duplicate (Autodesk Fusion 360 design; units mm, degrees)
Autodesk Fusion 360 part; units mm, degrees
sketch "Sketch2" plane through (0, 0, 0) normal (0, 1, 0) x (1, 0, 0) in component "oldroom"
  line L0 (0, 0) -> (2909, 0)
  line L1 (2909, 0) -> (2909, -3651)
  line L2 (2909, -3651) -> (0, -3651)
  line L3 (0, -3651) -> (0, 0)
  line L4 (2909, 0) -> (1648, 0)
  line L5 (1648, 0) -> (1648, -944)
  line L6 (1648, -944) -> (2909, -944)
  line L7 (2909, -944) -> (2909, 0)
  constraint horizontal L0
  constraint vertical L1
  constraint horizontal L2
  constraint vertical L3
  constraint coincident L0.start L3.end
  constraint horizontal L4
  constraint vertical L5
  constraint horizontal L6
  constraint vertical L7
extrude "Extrude1" add sketch "Sketch2" against normal blind 100 makes body 1 in component "walls"
extrude "Extrude2" add sketch "Sketch2" along normal blind 2405 contours L0 L1 L4 L5 L6 L7 bodies 1 in component "walls"
sketch "Sketch1" plane through (0, 0, 0) normal (0, 0, 1) x (1, 0, 0) in component "walls"
  line L0 (0, 0) -> (2909, 0)
  line L1 (2909, 0) -> (2909, 2405)
  line L2 (2909, 2405) -> (0, 2405)
  line L3 (0, 2405) -> (0, 0)
  line L4 (2909, -100) -> (2909, 2405)
  line L5 (2909, 0) -> (2909, 2405)
  constraint horizontal L0
  constraint vertical L1
  constraint horizontal L2
  constraint vertical L3
  constraint coincident L1.end L4
  constraint coincident L0.start L3.end
sketch "Sketch2 (2)" plane through (0, 0, 0) normal (1, 0, 0) x (0, 0, -1) in component "walls"
  line L0 (0, 0) -> (-3651, 0)
  line L1 (-3651, 0) -> (-3651, 2405)
  line L2 (-3651, 2405) -> (0, 2405)
  line L3 (0, 2405) -> (0, 0)
  constraint horizontal L0
  constraint vertical L1
  constraint horizontal L2
  constraint vertical L3
  constraint coincident L0.start L3.end
sketch "Sketch3" plane through (1648, 0, 0) normal (-1, 0, 0) x (0, 0, 1) in component "walls"
  line L0 (0, 0) -> (944, 0)
  line L1 (944, 0) -> (944, 2405)
  line L2 (944, 2405) -> (0, 2405)
  line L3 (0, 2405) -> (0, 0)
  line L4 (100, 0) -> (862, 0)
  line L5 (862, 0) -> (862, 1879.6)
  line L6 (862, 1879.6) -> (100, 1879.6)
  line L7 (100, 1879.6) -> (100, 0)
  constraint horizontal L4
  constraint vertical L5
  constraint horizontal L6
  constraint vertical L7
sketch "Sketch1 (2)" plane through (1648, 939.8, 481) normal (-1, 0, 0) x (0, 0, 1) in component "door"
extrude "Extrude1'" add sketch "Sketch3" against normal blind 35 separate body contours L0 L4 L5 L6 L7 makes body 2 in component "door"
sketch "Sketch1 (3)" plane through (0, 0, 0) normal (0, 1, 0) x (1, 0, 0) in component "shelving"
  line L0 (0, 0) -> (410, 0)
  line L1 (410, 0) -> (410, -910)
  line L2 (410, -910) -> (0, -910)
  line L3 (0, -910) -> (0, 0)
  constraint horizontal L0
  constraint vertical L1
  constraint horizontal L2
  constraint vertical L3
  constraint coincident L0.start L3.end
extrude "Extrude1''" add sketch "Sketch1 (3)" along normal blind 1830 separate body makes body 3 in component "shelving"
sketch "Sketch1 (4)" plane through (0, 0, 0) normal (0, 1, 0) x (1, 0, 0) in component "bed"
  line L0 (0, 0) -> (910, 0)
  line L1 (910, 0) -> (910, -1900)
  line L2 (910, -1900) -> (0, -1900)
  line L3 (0, -1900) -> (0, 0)
  constraint horizontal L0
  constraint vertical L1
  constraint horizontal L2
  constraint vertical L3
  constraint coincident L0.start L3.end
extrude "Extrude1'''" add sketch "Sketch1 (4)" along normal blind 800 separate body makes body 4 in component "bed"
move_body "Align1" bodies 4 to x (1, 0, 0) y (0, 1, 0) z (0, 0, 1) at (-146, 0, 0) in component "bed"
move_body "Align2" bodies 4 to x (1, 0, 0) y (0, 1, 0) z (0, 0, 1) at (0, 0, 4) in component "bed"
sketch "Sketch1 (5)" plane through (0, 0, 0) normal (0, 1, 0) x (1, 0, 0) in component "junk boxes"
  line L0 (2909, -3651) -> (1009, -3651)
  line L1 (1009, -3651) -> (1009, -2251)
  line L2 (1009, -2251) -> (2909, -2251)
  line L3 (2909, -2251) -> (2909, -3651)
  point P0 (2909, -3651)
  constraint horizontal L0
  constraint vertical L1
  constraint horizontal L2
  constraint vertical L3
  constraint coincident P0 L0.start
extrude "Extrude1''''" add sketch "Sketch1 (5)" along normal blind 200 separate body makes body 5 in component "junk boxes"
move_body "Align1'" bodies 3 to x (1, 0, 0) y (0, 1, 0) z (0, 0, 1) at (-31, 0, 0) in component "shelving"
move_face "MoveFace1" by (0, 0, -950) 1 faces at (2275.6667, 66.6667, 3651) on bodies 5 in component "junk boxes"
move_face "MoveFace2" by (0, 800, 0) 1 faces at (2275.6667, 200, 2551) on bodies 5 in component "junk boxes"
move_face "MoveFace3" by (1000, 0, 0) 1 faces at (1009, 333.3333, 2551) on bodies 5 in component "junk boxes"
sketch "Sketch1 (6)" plane through (0, 0, 0) normal (0, 1, 0) x (1, 0, 0) in component "computer table"
  line L0 (2909, -944) -> (2179, -944)
  line L1 (2179, -944) -> (2179, -1800)
  line L2 (2179, -1800) -> (2909, -1800)
  line L3 (2909, -1800) -> (2909, -944)
  point P0 (2909, -944)
  constraint horizontal L0
  constraint vertical L1
  constraint horizontal L2
  constraint vertical L3
  constraint coincident P0 L0.start
extrude "Extrude1'''''" add sketch "Sketch1 (6)" along normal blind 730 separate body makes body 6 in component "computer table"
sketch "Sketch1 (7)" plane through (0, 0, 0) normal (0, 1, 0) x (1, 0, 0) in component "chair"
  line L0 (1000, -1100) -> (1510, -1100)
  line L1 (1510, -1100) -> (1510, -1670)
  line L2 (1510, -1670) -> (1000, -1670)
  line L3 (1000, -1670) -> (1000, -1100)
  constraint horizontal L0
  constraint vertical L1
  constraint horizontal L2
  constraint vertical L3
extrude "Extrude1''''''" add sketch "Sketch1 (7)" along normal blind 560 separate body makes body 7 in component "chair"
sketch "Sketch2 (3)" plane through (0, 560, 0) normal (0, 1, 0) x (-1, 0, 0) in component "chair"
  line L0 (-1000, 1670) -> (-1510, 1670)
  line L1 (-1510, 1670) -> (-1510, 1100)
  line L2 (-1510, 1100) -> (-1000, 1100)
  line L3 (-1000, 1100) -> (-1000, 1670)
  line L4 (-1000, 1100) -> (-900, 1100)
  line L5 (-900, 1100) -> (-900, 1670)
  line L6 (-900, 1670) -> (-1000, 1670)
  line L7 (-1000, 1670) -> (-1000, 1100)
  constraint horizontal L4
  constraint vertical L5
  constraint horizontal L6
  constraint vertical L7
  constraint coincident L2.end L3.start
extrude "Extrude2'" add sketch "Sketch2 (3)" along normal blind 590 separate body contours L3 L4 L5 L6 L7 makes body 8 in component "chair"
sketch "Sketch1 (8)" plane through (0, 0, 0) normal (0, 1, 0) x (1, 0, 0) in component "small chest of draws"
  line L0 (0, -3651) -> (634.8984, -3651)
  line L1 (634.8984, -3651) -> (634.8984, -3214.5264)
  line L2 (634.8984, -3214.5264) -> (0, -3214.5264)
  line L3 (0, -3214.5264) -> (0, -3651)
  point P0 (0, -3651)
  constraint horizontal L0
  constraint vertical L1
  constraint horizontal L2
  constraint vertical L3
  constraint coincident P0 L0.start
extrude "Extrude1'''''''" add sketch "Sketch1 (8)" along normal blind 666.9024 separate body makes body 9 in component "small chest of draws"
sketch "Sketch1 (9)" plane through (0, 0, 0) normal (0, 1, 0) x (1, 0, 0) in component "wooden shelving"
  line L0 (0, 0) -> (500, 0)
  line L1 (500, 0) -> (500, -812)
  line L2 (500, -812) -> (0, -812)
  line L3 (0, -812) -> (0, 0)
  constraint horizontal L0
  constraint vertical L1
  constraint horizontal L2
  constraint vertical L3
  constraint coincident L0.start L3.end
extrude "Extrude1''''''''" add sketch "Sketch1 (9)" along normal blind 1800 separate body makes body 10 in component "wooden shelving"
sketch "Sketch1 (10)" plane through (0, 0, 0) normal (0, 1, 0) x (1, 0, 0) in component "chest of draws"
  line L0 (0, -800) -> (500, -800)
  line L1 (500, -800) -> (500, -1416)
  line L2 (500, -1416) -> (0, -1416)
  line L3 (0, -1416) -> (0, -800)
  constraint horizontal L0
  constraint vertical L1
  constraint horizontal L2
  constraint vertical L3
extrude "Extrude1'''''''''" add sketch "Sketch1 (10)" along normal blind 1300 separate body makes body 11 in component "chest of draws"
sketch "Sketch1 (11)" plane through (0, 0, 0) normal (0, 1, 0) x (1, 0, 0) in component "hollow stand"
  line L0 (0, -1416) -> (500, -1416)
  line L1 (500, -1416) -> (500, -2516)
  line L2 (500, -2516) -> (0, -2516)
  line L3 (0, -2516) -> (0, -1416)
  point P0 (0, -1416)
  constraint horizontal L0
  constraint vertical L1
  constraint horizontal L2
  constraint vertical L3
  constraint coincident P0 L0.start
extrude "Extrude1''''''''''" add sketch "Sketch1 (11)" along normal blind 910 separate body makes body 12 in component "hollow stand"
move_body "Align1''" bodies 11 to x (1, 0, 0) y (0, 1, 0) z (0, 0, 1) at (0, 0, 12) in component "chest of draws"
move_body "Align2'" bodies 11 to x (1, 0, 0) y (0, 1, 0) z (0, 0, 1) at (0, 0, -190) in component "chest of draws"
move_body "Align1'''" bodies 12 to x (1, 0, 0) y (0, 1, 0) z (0, 0, 1) at (0, 0, 12) in component "hollow stand"
move_body "Align2''" bodies 12 to x (1, 0, 0) y (0, 1, 0) z (0, 0, 1) at (0, 0, 0) in component "hollow stand"
move_body "Align3" bodies 12 to x (1, 0, 0) y (0, 1, 0) z (0, 0, 1) at (0, 0, -70) in component "hollow stand"
sketch "Sketch1 (12)" plane through (0, 0, 0) normal (0, 1, 0) x (1, 0, 0) in component "bed (1)"
  line L0 (0, 0) -> (910, 0)
  line L1 (910, 0) -> (910, -1900)
  line L2 (910, -1900) -> (0, -1900)
  line L3 (0, -1900) -> (0, 0)
  constraint horizontal L0
  constraint vertical L1
  constraint horizontal L2
  constraint vertical L3
  constraint coincident L0.start L3.end
extrude "Extrude1'''''''''''" add sketch "Sketch1 (12)" along normal blind 800 separate body makes body 13 in component "bed (1)"
move_body "Align1''''" bodies 13 to x (1, 0, 0) y (0, 1, 0) z (0, 0, 1) at (-146, 0, 0) in component "bed (1)"
move_body "Align2'''" bodies 13 to x (1, 0, 0) y (0, 1, 0) z (0, 0, 1) at (0, 0, 4) in component "bed (1)"
extrude "Extrude1''''''''''''" add 1 faces at (157.3333, 800, 1270.6667) faces seen with x (0, 0, -1) y (0, 1, 0) z (1, 0, 0) at (1005, 0, 3505) along direction (0, -1, 0) blind 800 separate body on bodies 13 makes body 14 in component "newroom"
extrude "Extrude2''" cut 1 faces at (2275.6667, 800, 3347.6667) along direction (0, -1, 0) blind 550 on bodies 14 bodies 14 in component "newroom"
sketch "Sketch1 (13)" plane through (0, -300, 0) normal (0, 1, 0) x (-1, 0, 0) in component "desk 1"
  line L0 (-1009, 4002.0003) -> (-65, 4002.0003)
  line L1 (-65, 4002.0003) -> (-65, 5650.0003)
  line L2 (-65, 5650.0003) -> (-3716, 5650.0003)
  line L3 (-3716, 5650.0003) -> (-3716, 2741.0003)
  line L4 (-3716, 2741.0003) -> (-1009, 2741.0003)
  line L5 (-1009, 2741.0003) -> (-1009, 4002.0003)
  line L6 (-65, 5650.0003) -> (-3716, 5650.0003)
  line L7 (-3716, 5650.0003) -> (-3716, 4750.0003)
  line L8 (-3716, 4750.0003) -> (-65, 4750.0003)
  line L9 (-65, 4750.0003) -> (-65, 5650.0003)
  constraint horizontal L6
  constraint vertical L7
  constraint horizontal L8
  constraint vertical L9
  constraint coincident L3 L7.end
  constraint coincident L1.end L2.start
extrude "Extrude1'''''''''''''" add sketch "Sketch1 (13)" along normal blind 50 separate body contours L1 L2 L3 L6 L7 L8 L9 makes body 15 in component "desk 1"
copy_body "CutPasteBodies1" bodies 14 removing the originals makes body 16 in component "bed (2)"
sketch "Sketch1 (14)" plane through (65, -300, 5650.0003) normal (0, 0, -1) x (-1, 0, 0) in component "Component"
sketch "Sketch2 (4)" plane through (0, -300, 0) normal (0, 1, 0) x (-1, 0, 0) in component "Component"
  line L0 (-1009, 4002.0003) -> (-65, 4002.0003)
  line L1 (-65, 4002.0003) -> (-65, 5650.0003)
  line L2 (-65, 5650.0003) -> (-3716, 5650.0003)
  line L3 (-3716, 5650.0003) -> (-3716, 2741.0003)
  line L4 (-3716, 2741.0003) -> (-1009, 2741.0003)
  line L5 (-1009, 2741.0003) -> (-1009, 4002.0003)
sketch "Sketch1 (15)" plane through (65, -300, 5650.0003) normal (0, 0, -1) x (-1, 0, 0) in component "lcd"
  line L0 (-2955.2121, 1965.6881) -> (-2314.4721, 1965.6881)
  line L1 (-2314.4721, 1965.6881) -> (-2314.4721, 1586.0281)
  line L2 (-2314.4721, 1586.0281) -> (-2955.2121, 1586.0281)
  line L3 (-2955.2121, 1586.0281) -> (-2955.2121, 1965.6881)
  constraint horizontal L0
  constraint vertical L1
  constraint horizontal L2
  constraint vertical L3
extrude "Extrude1''''''''''''''" add sketch "Sketch1 (15)" along normal blind 51.5 separate body makes body 17 in component "lcd"
copy_body "CopyPasteBodies1" bodies 17 makes body 18 in component "lcd"
move_body "Move1" bodies 18 to x (1, 0, 0) y (0, 1, 0) z (0, 0, 1) at (-700, 0, 0) in component "lcd"
sketch "Sketch2 (5)" plane through (465, 200, 5650.0003) normal (0, 0, -1) x (-1, 0, 0) in component "lcd"
  line L0 (-1914.4721, 1465.6881) -> (-1855.2121, 1465.6881)
  line L1 (-1855.2121, 1465.6881) -> (-1855.2121, 850.1808)
  line L2 (-1855.2121, 850.1808) -> (-1914.4721, 850.1808)
  line L3 (-1914.4721, 850.1808) -> (-1914.4721, 1465.6881)
  line L4 (-1855.2121, 1359.1726) -> (-1535.2121, 1359.1726)
  line L5 (-1535.2121, 1359.1726) -> (-1535.2121, 1259.1726)
  line L6 (-1535.2121, 1259.1726) -> (-1855.2121, 1259.1726)
  line L7 (-1855.2121, 1259.1726) -> (-1855.2121, 1359.1726)
  line L8 (-1914.4721, 1359.1726) -> (-2234.4721, 1359.1726)
  line L9 (-2234.4721, 1359.1726) -> (-2234.4721, 1259.1726)
  line L10 (-2234.4721, 1259.1726) -> (-1914.4721, 1259.1726)
  line L11 (-1914.4721, 1259.1726) -> (-1914.4721, 1359.1726)
  point P0 (-1914.4721, 1465.6881)
  constraint horizontal L0
  constraint vertical L1
  constraint horizontal L2
  constraint vertical L3
  constraint coincident P0 L0.start
  constraint horizontal L4
  constraint vertical L5
  constraint horizontal L6
  constraint vertical L7
  constraint coincident L1 L4.start
  constraint horizontal L8
  constraint vertical L9
  constraint horizontal L10
  constraint vertical L11
  constraint coincident L3 L8.start
extrude "Extrude2'''" add sketch "Sketch2 (5)" along normal blind 100 separate body makes body 19 in component "lcd"
extrude "Extrude3" cut 1 faces at (2592.8054, 1492.5059, 5550.0003) along direction (0, 0, 1) blind 50 on bodies 19 bodies 17 18 19 in component "lcd"
move_body "Move2" bodies 17 18 to x (1, 0, 0) y (0, 1, 0) z (0, 0, 1) at (0, 0, -100) in component "lcd"
combine "Combine1" operation add target body 17 tool bodies 19 makes body 20 at (2592.8054, 1492.5059, 5650.0003) in component "lcd"
extrude "Extrude4" add 1 faces at (2213.5454, 1525.8393, 5500.0003) along direction (0, 0, -1) blind 1 on bodies 18 bodies 18 in component "lcd"
extrude "Extrude5" add 1 faces at (2213.5454, 1525.8393, 5499.0003) along direction (0, 0, -1) blind 0.5 on bodies 18 bodies 18 in component "lcd"
extrude "Extrude6" add 1 faces at (2592.8054, 1492.5059, 5500.0003) along direction (0, 0, -1) blind 1.5 on bodies 17 bodies 17 in component "lcd"
sketch "Sketch1 (16)" plane through (0, -300, 0) normal (0, 1, 0) x (-1, 0, 0) in component "AC"
  line L0 (-3500, 4500) -> (-3035, 4500)
  line L1 (-3035, 4500) -> (-3035, 4100)
  line L2 (-3035, 4100) -> (-3500, 4100)
  line L3 (-3500, 4100) -> (-3500, 4500)
  constraint horizontal L0
  constraint vertical L1
  constraint horizontal L2
  constraint vertical L3
extrude "Extrude1'''''''''''''''" add sketch "Sketch1 (16)" along normal blind 765 separate body makes body 21 in component "AC"
sketch "Sketch1 (17)" plane through (65, -300, 5650.0003) normal (0, 0, -1) x (-1, 0, 0) in component "lcd (1)"
  line L0 (-2955.2121, 1965.6881) -> (-2314.4721, 1965.6881)
  line L1 (-2314.4721, 1965.6881) -> (-2314.4721, 1586.0281)
  line L2 (-2314.4721, 1586.0281) -> (-2955.2121, 1586.0281)
  line L3 (-2955.2121, 1586.0281) -> (-2955.2121, 1965.6881)
  constraint horizontal L0
  constraint vertical L1
  constraint horizontal L2
  constraint vertical L3
extrude "Extrude1''''''''''''''''" add sketch "Sketch1 (17)" along normal blind 51.5 separate body makes body 22 in component "lcd (1)"
copy_body "CopyPasteBodies1'" bodies 22 makes body 23 in component "lcd (1)"
move_body "Move1'" bodies 23 to x (1, 0, 0) y (0, 1, 0) z (0, 0, 1) at (-700, 0, 0) in component "lcd (1)"
sketch "Sketch2 (6)" plane through (465, 200, 5650.0003) normal (0, 0, -1) x (-1, 0, 0) in component "lcd (1)"
  line L0 (-1914.4721, 1465.6881) -> (-1855.2121, 1465.6881)
  line L1 (-1855.2121, 1465.6881) -> (-1855.2121, 850.1808)
  line L2 (-1855.2121, 850.1808) -> (-1914.4721, 850.1808)
  line L3 (-1914.4721, 850.1808) -> (-1914.4721, 1465.6881)
  line L4 (-1855.2121, 1359.1726) -> (-1535.2121, 1359.1726)
  line L5 (-1535.2121, 1359.1726) -> (-1535.2121, 1259.1726)
  line L6 (-1535.2121, 1259.1726) -> (-1855.2121, 1259.1726)
  line L7 (-1855.2121, 1259.1726) -> (-1855.2121, 1359.1726)
  line L8 (-1914.4721, 1359.1726) -> (-2234.4721, 1359.1726)
  line L9 (-2234.4721, 1359.1726) -> (-2234.4721, 1259.1726)
  line L10 (-2234.4721, 1259.1726) -> (-1914.4721, 1259.1726)
  line L11 (-1914.4721, 1259.1726) -> (-1914.4721, 1359.1726)
  point P0 (-1914.4721, 1465.6881)
  constraint horizontal L0
  constraint vertical L1
  constraint horizontal L2
  constraint vertical L3
  constraint coincident P0 L0.start
  constraint horizontal L4
  constraint vertical L5
  constraint horizontal L6
  constraint vertical L7
  constraint coincident L1 L4.start
  constraint horizontal L8
  constraint vertical L9
  constraint horizontal L10
  constraint vertical L11
  constraint coincident L3 L8.start
extrude "Extrude2''''" add sketch "Sketch2 (6)" along normal blind 100 separate body makes body 24 in component "lcd (1)"
extrude "Extrude3'" cut 1 faces at (2592.8054, 1492.5059, 5550.0003) along direction (0, 0, 1) blind 50 on bodies 24 bodies 22 23 24 in component "lcd (1)"
move_body "Move2'" bodies 22 23 to x (1, 0, 0) y (0, 1, 0) z (0, 0, 1) at (0, 0, -100) in component "lcd (1)"
combine "Combine1'" operation add target body 22 tool bodies 24 makes body 25 at (2592.8054, 1492.5059, 5650.0003) in component "lcd (1)"
extrude "Extrude4'" add 1 faces at (2213.5454, 1525.8393, 5500.0003) along direction (0, 0, -1) blind 1 on bodies 23 bodies 23 in component "lcd (1)"
extrude "Extrude5'" add 1 faces at (2213.5454, 1525.8393, 5499.0003) along direction (0, 0, -1) blind 0.5 on bodies 23 bodies 23 in component "lcd (1)"
extrude "Extrude6'" add 1 faces at (2592.8054, 1492.5059, 5500.0003) along direction (0, 0, -1) blind 1.5 on bodies 22 bodies 22 in component "lcd (1)"
move_body "Move3" bodies 22 to x (1, 0, 0) y (0, 1, 0) z (0, 0, 1) at (-60, 0, 0) in component "lcd (1)"
move_body "Move4" bodies 25 to x (1, 0, 0) y (0, 1, 0) z (0, 0, 1) at (-30, 0, 0) in component "lcd (1)"
component "walls" placed x (1, 0, 0) y (0, 1, 0) z (0, 0, 1) at (0, 0, 0)
component "oldroom" placed x (1, 0, 0) y (0, 1, 0) z (0, 0, 1) at (0, 0, 0)
component "newroom" placed x (0, 0, 1) y (0, 1, 0) z (-1, 0, 0) at (5650.0003, 300, -65)
component "junk boxes" placed x (1, 0, 0) y (0, 1, 0) z (0, 0, 1) at (-900, 0, 950) in component "oldroom"
component "bed" placed x (1, 0, 0) y (0, 1, 0) z (0, 0, 1) at (2145, 0, 940) in component "oldroom"
component "computer table" placed x (0, 0, 1) y (0, 1, 0) z (-1, 0, 0) at (1816, 0, 728) in component "oldroom"
component "chair" placed x (0, 0, 1) y (0, 1, 0) z (-1, 0, 0) at (1840, 0, 1530) in component "oldroom"
component "small chest of draws" placed x (1, 0, 0) y (0, 1, 0) z (0, 0, 1) at (0, 0, 1100) in component "oldroom"
component "wooden shelving" placed x (1, 0, 0) y (0, 1, 0) z (0, 0, 1) at (0, 0, 0) in component "oldroom"
component "chest of draws" placed x (1, 0, 0) y (0, 1, 0) z (0, 0, 1) at (0, 0, 190) in component "oldroom"
component "hollow stand" placed x (0, 0, -1) y (0, 1, 0) z (1, 0, 0) at (-1358, 0, 3651) in component "oldroom"
component "shelving" placed x (0, 0, -1) y (0, 1, 0) z (1, 0, 0) at (2000, 0, 3620) in component "oldroom"
component "lcd (1)" placed x (1, 0, 0) y (0, 1, 0) z (0, 0, 1) at (-1674.2489, -199.9801, -2089.1804) in component "oldroom"
component "door" placed x (1, 0, 0) y (0, 1, 0) z (0, 0, 1) at (-20, 0, 0) in component "walls"
component "desk 1" placed x (1, 0, 0) y (0, 1, 0) z (0, 0, 1) at (0, 800, 0) in component "newroom"
component "bed (2)" placed x (1, 0, 0) y (0, 1, 0) z (0, 0, 1) at (0, 0, 0) in component "newroom"
component "Component" placed x (1, 0, 0) y (0, 1, 0) z (0, 0, 1) at (0, 0, 0) in component "newroom"
component "chair" placed x (0, 0, 1) y (0, 1, 0) z (-1, 0, 0) at (3405, -300, 3350.0003) in component "newroom"
component "lcd" placed x (1, 0, 0) y (0, 1, 0) z (0, 0, 1) at (-399.7722, -499.9801, 0.1568) in component "newroom"
component "AC" placed x (1, 0, 0) y (0, 1, 0) z (0, 0, 1) at (0, 0, 950.0003) in component "newroom"
equation "d10 = 2'-0\" + 6\""
equation "d11 = 6'-0\" + 2\""
equation "d84 = 5.000E-04 m"
equation "d84_1 = 5.000E-04 m"
